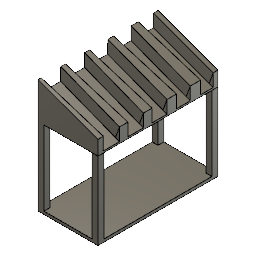
rail_interieur v3 (Autodesk Fusion 360 design; units mm, degrees)
Autodesk Fusion 360 part; units mm, degrees
note: some values were not read from the file. Chosen so that the rebuilt part matches the saved one: which pieces of a blend or face edit are solid.
sketch "Sketch1" plane through (0, 0, 0) normal (0, 0, 1) x (1, 0, 0)
  line L0 (0, 0) -> (100, 0)
  line L1 (100, 0) -> (100, 76)
  line L2 (100, 76) -> (0, 76)
  line L3 (0, 76) -> (0, 0)
  dimension "d17" = 76
  dimension "d18" = 100
  measures "d17" distance of L0.start
  measures "d18" distance of L0.start
extrude "Extrude1" add sketch "Sketch1" along normal blind 200
sketch "Sketch2" plane through (0, 0, 0) normal (0, 0, -1) x (-1, 0, 0)
  line L0 (0, 0) -> (0, 76)
  line L1 (0, 76) -> (-100, 76)
  line L2 (-100, 76) -> (-100, 0)
  line L3 (-100, 0) -> (0, 0)
  line L4 (0, 76) -> (0, 29.8312)
  line L5 (-100, 39.603) -> (0, 76)
  line L6 (-100, 39.603) -> (0, 29.8312)
  dimension "d21" = 70
  measures "d21" angle of L4 L5
extrude "Extrude2" cut sketch "Sketch2" against normal blind 200 contours L1 L2 L5
sketch "Sketch3" plane through (24.4259, 67.1097, 0) normal (0.34202, 0.939693, 0) x (0, 0, -1)
  line L0 (0, -80.4242) -> (0, 25.9935)
  line L1 (0, 25.9935) -> (-200, 25.9935)
  line L2 (-200, 25.9935) -> (-200, -80.4242)
  line L3 (-200, -80.4242) -> (0, -80.4242)
  line L4 (-194.57, 25.9935) -> (-162.27, 25.9935)
  line L5 (-164.07, -80.4242) -> (-162.27, 25.9935)
  line L6 (-194.57, 25.9935) -> (-191.07, -80.4242)
  line L7 (-164.07, -80.4242) -> (-191.07, -80.4242)
  line L8 (-154.33, 25.9935) -> (-122.33, 25.9935)
  line L9 (-124.2, -80.4242) -> (-122.33, 25.9935)
  line L10 (-154.33, 25.9935) -> (-150.2, -80.4242)
  line L11 (-113.93, 25.9935) -> (-83.93, 25.9935)
  line L12 (-84.95, -80.4242) -> (-109.95, -80.4242)
  line L13 (-113.93, 25.9935) -> (-109.95, -80.4242)
  line L14 (-83.93, 25.9935) -> (-84.95, -80.4242)
  line L15 (-69.2, -80.4242) -> (-73.98, 25.9935)
  line L16 (-73.98, 25.9935) -> (-44.98, 25.9935)
  line L17 (-44.98, 25.9935) -> (-46.2, -80.4242)
  line L18 (-69.2, -80.4242) -> (-46.2, -80.4242)
  line L19 (-29, -80.4242) -> (-32.78, 25.9935)
  line L20 (-7.78, 25.9935) -> (-32.78, 25.9935)
  line L21 (-7.78, 25.9935) -> (-8, -80.4242)
  line L22 (-29, -80.4242) -> (-8, -80.4242)
  dimension "d24" = 7.78
  dimension "d25" = 25
  dimension "d26" = 21
  dimension "d27" = 8
  dimension "d28" = 12.2
  dimension "d29" = 29
  dimension "d30" = 23
  dimension "d31" = 17.2
  dimension "d32" = 9.95
  dimension "d33" = 30
  dimension "d34" = 15.75
  dimension "d35" = 25
  dimension "d36" = 8.4
  dimension "d37" = 32
  dimension "d38" = 14.25
  dimension "d39" = 26
  dimension "d40" = 13.87
  dimension "d41" = 32.3
  dimension "d42" = 7.94
  dimension "d43" = 27
  measures "d24" distance of origin
  measures "d25" distance of origin
  measures "d26" distance of origin
  measures "d27" distance of origin
extrude "Extrude3" cut sketch "Sketch3" against normal blind 20 contours L1 L3 L19 L20 L21 L22 | L1 L3 L15 L16 L17 L18 | L1 L3 L11 L12 L13 L14 | L1 L3 L8 L9 L10 | L1 L3 L4 L5 L6 L7
extrude "Extrude4" cut 5 faces at (95.4397, 27.0737, 101.6167) (97.7199, 33.3384, 141.5333) (95.4397, 27.0737, 182.07) (97.7199, 33.3384, 53.8667) (97.7199, 33.3384, 22) along direction (0.939693, -0.34202, 0) blind 20
sketch "Sketch5" plane through (0, 0, 0) normal (0, 0, -1) x (-1, 0, 0)
  line L0 (0, 76) -> (-100, 39.603)
  line L1 (-100, 39.603) -> (-100, 0)
  line L2 (-100, 0) -> (0, 0)
  line L3 (0, 0) -> (0, 76)
  line L4 (-100, 0) -> (0, 0)
  line L5 (0, 0) -> (0, 15.3194)
  line L6 (0, 15.3194) -> (-100, 15.3194)
  line L7 (-100, 15.3194) -> (-100, 0)
  dimension "d48" = 3
extrude "Extrude5" cut sketch "Sketch5" against normal blind 200 contours L1 L2 L3 L4 L5 L6 L7
sketch "Sketch7" plane through (0, 0, 0) normal (0, 1, 0) x (1, 0, 0)
  line L0 (100, -8) -> (100, -29)
  line L1 (0, -7.78) -> (100, -8)
  circle A0 centre (110.5, -18.5231) radius 10.5
  line L2 (0, -44.98) -> (100, -46.2)
  line L3 (100, -46.2) -> (100, -69.2)
  circle A1 centre (111.5, -57.8412) radius 11.5
  line L4 (0, -83.93) -> (100, -84.95)
  line L5 (100, -84.95) -> (100, -109.95)
  circle A2 centre (112.5, -97.5782) radius 12.5
  line L6 (0, -122.33) -> (100, -124.2)
  line L7 (100, -124.2) -> (100, -150.2)
  circle A3 centre (113, -137.4454) radius 13
  line L8 (0, -162.27) -> (100, -164.07)
  line L9 (100, -164.07) -> (100, -191.07)
  circle A4 centre (113.5, -177.8152) radius 13.5
  circle A5 centre (113.5, -177.8152) radius 15.5
  circle A6 centre (113, -137.4454) radius 15
  circle A7 centre (112.5, -97.5782) radius 14.5
  circle A8 centre (111.5, -57.8412) radius 13.5
  circle A9 centre (110.5, -18.5231) radius 12.5
  dimension "d51" = 21
  dimension "d52" = 23
  dimension "d53" = 25
  dimension "d54" = 26
  dimension "d55" = 27
  dimension "d56" = 2
  dimension "d57" = 2
  dimension "d58" = 2
  dimension "d59" = 2
  dimension "d60" = 2
  measures "d51" diameter of A0
  measures "d52" diameter of A1
  measures "d53" diameter of A2
  measures "d54" diameter of A3
  measures "d55" diameter of A4
  measures "d56" distance of A4 A5
  measures "d57" distance of A3 A6
  measures "d58" distance of A2 A7
  measures "d59" distance of A1 A8
  measures "d60" distance of A0 A9
sketch "Sketch8" plane through (0, 0, 200) normal (0, 0, 1) x (1, 0, 0)
  line L0 (0, 15.3194) -> (100, 15.3194)
  line L1 (100, 15.3194) -> (100, 39.603)
  line L2 (100, 39.603) -> (0, 76)
  line L3 (0, 76) -> (0, 15.3194)
  line L4 (0, 95) -> (39.9891, 61.4452)
  line L5 (0, 76) -> (0, 95)
  line L6 (0, 76) -> (39.9891, 61.4452)
  dimension "d65" = 50
  measures "d65" angle of L4 L5
sketch "Sketch9" plane through (-2.5854, 0.941, 162.6631) normal (-0.015892, 0.005784, 0.999857) x (0.999874, 0, 0.015892)
  line L0 (2.5789, 75.0602) -> (2.5808, 53.7763)
  line L1 (2.5808, 53.7763) -> (95.7553, 19.8684)
  line L2 (95.7553, 19.8684) -> (102.5948, 38.6626)
  line L3 (102.5948, 38.6626) -> (2.5789, 75.0602)
  line L4 (3.1785, 93.8417) -> (43.1625, 60.2911)
  line L5 (3.1785, 74.842) -> (3.1785, 93.8417)
  line L6 (3.1785, 74.842) -> (43.1625, 60.2911)
sketch "Sketch17" plane through (100, 0, 0) normal (-1, 0, 0) x (0, 0, 1)
  line L0 (177.8152, -5) -> (177.8152, 15.319)
  line L1 (177.8152, 15.319) -> (170.1994, 15.319)
  line L2 (170.1994, 15.319) -> (170.1994, -5)
  line L3 (170.1994, -5) -> (177.8152, -5)
  line L4 (185.431, -5) -> (11.7408, -5)
  line L5 (11.7408, -5) -> (11.7408, 15.319)
  line L6 (11.7408, 15.319) -> (185.431, 15.319)
  line L7 (185.431, 15.319) -> (185.431, -5)
  line L8 (11.7408, -5) -> (11.7408, 15.319)
  line L9 (200, 15.3194) -> (0, 15.3194)
  line L10 (137.4454, -5) -> (137.4454, 15.319)
  line L11 (137.4454, 15.319) -> (129.9621, 15.319)
  line L12 (129.9621, 15.319) -> (129.9621, -5)
  line L13 (129.9621, -5) -> (137.4454, -5)
sketch "Sketch18" plane through (100, 0, 0) normal (1, 0, 0) x (0, 0, -1)
  line L0 (-185.431, -5) -> (-11.7408, -5)
  line L1 (-11.7408, 15.319) -> (-185.431, 15.319)
  line L2 (-129.9621, -5) -> (-129.9621, 15.319)
  line L3 (-122.4454, 15.319) -> (-152.4454, 15.319)
  line L4 (-144.9287, 15.319) -> (-144.9287, -5)
  line L5 (-152.4454, -5) -> (-122.4454, -5)
  line L6 (-170.1994, -5) -> (-170.1994, 15.319)
  line L7 (-162.3152, 15.319) -> (-193.3152, 15.319)
  line L8 (-185.431, 15.319) -> (-185.431, -5)
  line L9 (-193.3152, -5) -> (-162.3152, -5)
  line L10 (-90.2297, -5) -> (-90.2297, 15.319)
  line L11 (-83.0782, 15.319) -> (-112.0782, 15.319)
  line L12 (-104.9266, 15.319) -> (-104.9266, -5)
  line L13 (-112.0782, -5) -> (-83.0782, -5)
  line L14 (-50.7701, -5) -> (-50.7701, 15.319)
  line L15 (-44.3412, 15.319) -> (-71.3412, 15.319)
  line L16 (-64.9122, 15.319) -> (-64.9122, -5)
  line L17 (-71.3412, -5) -> (-44.3412, -5)
  line L18 (-11.7408, -5) -> (-11.7408, 15.319)
  line L19 (-6.0231, 15.319) -> (-31.0231, 15.319)
  line L20 (-25.3055, 15.319) -> (-25.3055, -5)
  line L21 (-31.0231, -5) -> (-6.0231, -5)
  line L22 (-162.3152, 15.319) -> (-152.4454, 15.319)
  line L23 (-152.4454, 15.319) -> (-152.4454, -5)
  line L24 (-152.4454, -5) -> (-162.3152, -5)
  line L25 (-162.3152, -5) -> (-162.3152, 15.319)
  line L26 (-122.4454, 15.319) -> (-112.0782, 15.319)
  line L27 (-112.0782, 15.319) -> (-112.0782, -5)
  line L28 (-112.0782, -5) -> (-122.4454, -5)
  line L29 (-122.4454, -5) -> (-122.4454, 15.319)
  line L30 (-83.0782, 15.319) -> (-71.3412, 15.319)
  line L31 (-71.3412, 15.319) -> (-71.3412, -5)
  line L32 (-71.3412, -5) -> (-83.0782, -5)
  line L33 (-83.0782, -5) -> (-83.0782, 15.319)
  line L34 (-44.3412, 15.319) -> (-31.0231, 15.319)
  line L35 (-31.0231, 15.319) -> (-31.0231, -5)
  line L36 (-31.0231, -5) -> (-44.3412, -5)
  line L37 (-44.3412, -5) -> (-44.3412, 15.319)
  line L38 (-11.7408, -5) -> (-11.7408, 15.319)
  line L39 (-185.431, 15.319) -> (-185.431, -5)
sketch "Sketch19" plane through (0, 0, 0) normal (0, 0, -1) x (-1, 0, 0)
  line L0 (-100, 15.3194) -> (0, 15.3194)
  line L1 (0, 15.3194) -> (0, 76)
  line L2 (0, 76) -> (-100, 39.603)
  line L3 (-100, 39.603) -> (-100, 15.3194)
  line L4 (-10, 72.3603) -> (0, 76)
  line L5 (0, -114) -> (-10, -114)
  line L6 (-10, -114) -> (-10, 72.3603)
  line L7 (0, 76) -> (0, -114)
  dimension "d83" = 190
  dimension "d85" = 10
extrude "Extrude15" add sketch "Sketch19" against normal blind 10 contours L0 L5 L6 L7
sketch "Sketch20" plane through (0, 0, 200) normal (0, 0, 1) x (1, 0, 0)
  line L0 (0, 15.3194) -> (100, 15.3194)
  line L1 (100, 15.3194) -> (100, 39.603)
  line L2 (100, 39.603) -> (0, 76)
  line L3 (0, 76) -> (0, 15.3194)
  line L4 (10, -114) -> (10, 15.3194)
  line L5 (10, 15.3194) -> (0, 15.3194)
  line L6 (0, 15.3194) -> (0, -114)
  line L7 (0, -114) -> (10, -114)
extrude "Extrude16" add sketch "Sketch20" against normal blind 10 contours L0 L4 L5 L6 L7
sketch "Sketch21" plane through (0, -114, 0) normal (0, -1, 0) x (1, 0, 0)
  line L0 (10, 200) -> (0, 200)
  line L1 (0, 200) -> (0, 190)
  line L2 (0, 190) -> (10, 190)
  line L3 (10, 190) -> (10, 200)
  line L4 (0, 200) -> (100, 200)
  line L5 (100, 200) -> (100, 0)
  line L6 (100, 0) -> (0, 0)
  line L7 (0, 0) -> (0, 200)
  line L8 (10, 0) -> (10, 10)
  line L9 (0, 10) -> (10, 10)
extrude "Extrude17" add sketch "Sketch21" against normal blind 5 contours L2 L3 L4 L5 L6 L7 L8 L9
sketch "Sketch22" plane through (0, -109, 0) normal (0, 1, 0) x (-1, 0, 0)
  line L0 (0, 10) -> (0, 190)
  line L1 (0, 190) -> (-10, 190)
  line L2 (-10, 190) -> (-10, 200)
  line L3 (-10, 200) -> (-100, 200)
  line L4 (-100, 200) -> (-100, 0)
  line L5 (-100, 0) -> (-10, 0)
  line L6 (-10, 0) -> (-10, 10)
  line L7 (-10, 10) -> (0, 10)
  line L8 (-100, 200) -> (-90, 200)
  line L9 (-90, 200) -> (-90, 190)
  line L10 (-90, 190) -> (-100, 190)
  line L11 (-100, 190) -> (-100, 200)
  line L12 (-100, 0) -> (-90, 0)
  line L13 (-90, 0) -> (-90, 10)
  line L14 (-90, 10) -> (-100, 10)
  line L15 (-100, 10) -> (-100, 0)
  dimension "d92" = 10
  dimension "d93" = 10
  dimension "d94" = 10
  dimension "d95" = 10
  measures "d94" distance of origin L14
extrude "Extrude18" add sketch "Sketch22" along normal blind 124.319 contours L4 L5 L12 L13 L14 L15 | L3 L4 L8 L9 L10 L11
sketch "Sketch23" plane through (0, 0, 0) normal (0, 0, -1) x (-1, 0, 0)
  line L0 (-100, 15.3194) -> (-10, 15.3194)
  line L1 (-10, 15.3194) -> (-10, -109)
  line L2 (-10, -109) -> (-90, -109)
  line L3 (-90, -109) -> (-90, 15.319)
  line L4 (-90, 15.319) -> (-100, 15.319)
  line L5 (-100, 15.319) -> (-100, -114)
  line L6 (-100, -114) -> (0, -114)
  line L7 (0, -114) -> (0, 76)
  line L8 (0, 76) -> (-100, 39.603)
  line L9 (-100, 39.603) -> (-100, 15.3194)
  line L10 (0, 54.7164) -> (-93.1596, 20.8091)
  line L11 (-82.5201, 15.319) -> (0, 50)
  line L12 (0, 15.3194) -> (-82.5201, 15.319)
  line L13 (0, 50) -> (0, 15.3194)
ref_plane "WorkPlane1" through (128.9986, 8.5909, 177.6099) normal (0.999912, 0, -0.013244) x (0.013244, 0, 0.999912)
sketch "Sketch28" plane through (128.9986, 8.5909, 177.6099) normal (0.999912, 0, -0.013244) x (0.013244, 0, 0.999912)
  line L0 (-169.3037, -6.7285) -> (-169.3037, 117.5909)
  line L1 (-169.1713, 117.5909) -> (-169.1713, -6.7285)
  line L2 (-169.3037, 23.5909) -> (-169.1713, 28.5909)
  line L3 (40.1619, 65.502) -> (40.0294, 60.502)
  line L4 (40.0294, 60.502) -> (-169.3037, 23.5909)
  line L5 (-169.1713, 28.5909) -> (40.1619, 65.502)
  line L6 (-146.8178, 13.5909) -> (-171.8178, 13.5909)
  dimension "d107" = 100
  dimension "d108" = 5
  dimension "d109" = 5
  dimension "d110" = 10
  measures "d107" angle of L1 L4
  measures "d110" distance of origin L6
extrude "Extrude23" add sketch "Sketch28" against normal blind 28.147 contours L1 L3 L4 L5
ref_plane "WorkPlane2" through (50, -64, 100) normal (0, -1, 0) x (1, 0, 0)
sketch "Sketch30" plane through (50, -64, 100) normal (0, -1, 0) x (1, 0, 0)
  line L0 (50, -90) -> (50, -91.1921)
  line L1 (50, -91.1921) -> (76.7581, -91.5465)
  line L2 (76.7581, -91.5465) -> (79.5306, 117.7683)
  line L3 (79.5306, 117.7683) -> (51.386, 118.1411)
  line L4 (51.386, 118.1411) -> (48.6291, -90)
  line L5 (48.6291, -90) -> (50, -90)
  line L6 (76.7581, -91.5465) -> (66.8905, -91.4158)
  line L7 (66.8905, -81.4158) -> (76.8905, -81.5465)
  line L8 (76.7581, -91.5465) -> (76.8905, -81.5465)
  line L9 (66.8905, -81.4158) -> (66.8905, -91.4158)
  line L10 (79.5306, 117.7683) -> (79.3999, 107.9007)
  line L11 (69.3999, 107.9007) -> (69.5323, 117.9007)
  line L12 (79.5306, 117.7683) -> (69.5323, 117.9007)
  line L13 (69.3999, 107.9007) -> (79.3999, 107.9007)
  line L14 (51.386, 118.1411) -> (51.2536, 108.1428)
  line L15 (51.2536, 108.1428) -> (61.2536, 108.0104)
  line L16 (61.2536, 118.0104) -> (51.386, 118.1411)
  line L17 (61.2536, 108.0104) -> (61.2536, 118.0104)
  dimension "d120" = 10
  dimension "d121" = 10
  dimension "d122" = 10
  dimension "d123" = 10
  dimension "d124" = 10
  dimension "d125" = 10
  dimension "d126" = 10
extrude "Extrude24" add sketch "Sketch30" along normal blind 50 and the other way up to surface contours L1 L2 L6 L7 L8 L9 | L3 L4 L14 L15 L16 L17 | L2 L3 L10 L11 L12 L13 second end surface through (126.7581, -20, 8.4535) normal (-0.0023, -0.984808, -0.173633) offset 0
sketch "Sketch32" plane through (126.6239, 0, -1.6772) normal (0.999912, 0, -0.013244) x (-0.013244, 0, -0.999912)
  line L0 (-10.1316, -114) -> (-10.1316, -15.0234)
  line L1 (-10.1316, -15.0234) -> (-219.3323, -51.9111)
  line L2 (-219.3323, -51.9111) -> (-219.4647, -56.9111)
  line L3 (-219.4647, -56.9111) -> (-219.4647, -114)
  line L4 (-219.4647, -114) -> (-209.5963, -114)
  line L5 (-209.5963, -114) -> (-209.5963, -55.171)
  line L6 (-209.5963, -55.171) -> (-20.1324, -21.7634)
  line L7 (-20.1324, -21.7634) -> (-20.1324, -114)
  line L8 (-20.1324, -114) -> (-10.1316, -114)
  line L9 (-219.3323, -51.9111) -> (-159.9903, -41.4475)
  line L10 (-191.3078, -109) -> (-191.3078, 15.319)
  line L11 (-11.3236, -15.2335) -> (-10.1316, -15.0234)
  line L12 (-10.1316, -15.0234) -> (-10.1316, -20)
  line L13 (-10.1316, -20) -> (-11.3236, -20.2102)
  line L14 (-11.3236, -20.2102) -> (-11.3236, -109)
  line L15 (-11.3236, -109) -> (-191.3078, -109)
  line L16 (-191.3078, -109) -> (-191.3078, 15.319)
  line L17 (-191.3078, 15.319) -> (-201.3069, 15.319)
  line L18 (-201.3069, 15.319) -> (-201.3069, -114)
  line L19 (-201.3069, -114) -> (-1.3244, -114)
  line L20 (-1.3244, -114) -> (-1.3244, 15.319)
  line L21 (-1.3244, 15.319) -> (-11.3236, 15.319)
  line L22 (-11.3236, 15.319) -> (-11.3236, -15.2335)
extrude "Extrude25" add sketch "Sketch32" along normal up to surface contours L1 L6 L9 L10 L16 L18 end surface through (100, -114, 200) normal (1, 0, 0) offset 0
delete_face "DeleteFace1" 1 faces at (119.1, -37.968, 138.692)
extrude "Extrude19" [suppressed]
extrude "Extrude20" [suppressed]
sketch "Sketch25" plane through (0, 0, 0) normal (0, 0, -1) x (-1, 0, 0)
  line L0 (-10.0002, 45.7972) -> (-10, 15.3194)
  line L1 (-10, 15.3194) -> (-10, -109)
  line L2 (-10, -109) -> (-90, -109)
  line L3 (-90, -109) -> (-90, 15.319)
  line L4 (-90, 15.319) -> (-100, 15.319)
  line L5 (-100, 15.319) -> (-100, -114)
  line L6 (-100, -114) -> (0, -114)
  line L7 (0, -114) -> (0, 15.3194)
  line L8 (0, 15.3194) -> (-0.0002, 47.5734)
  line L9 (-0.0002, 47.5734) -> (-5.7739, 47.5734)
  line L10 (-5.7739, 47.5734) -> (0, 50)
  line L11 (0, 50) -> (0, 76)
  line L12 (0, 76) -> (-100, 39.603)
  line L13 (-100, 39.603) -> (-100, 15.3194)
  line L14 (-100, 15.3194) -> (-82.5191, 15.3194)
  line L15 (-82.5191, 15.3194) -> (-10.0002, 45.7972)
  line L16 (-5.7739, 47.5734) -> (0, 50)
  line L17 (0, 50) -> (-0.0002, 47.5734)
  line L18 (-0.0002, 47.5734) -> (-5.7739, 47.5734)
sketch "Sketch26" plane through (0, 0, 190) normal (0, 0, -1) x (-1, 0, 0)
  line L0 (-10, 15.3194) -> (-10, -109)
  line L1 (-10, -109) -> (0, -109)
  line L2 (0, -109) -> (0, 15.3194)
  line L3 (0, 15.3194) -> (-0.0002, 47.5734)
  line L4 (-0.0002, 47.5734) -> (-5.7739, 47.5734)
  line L5 (-5.7739, 47.5734) -> (-10.0002, 45.7972)
  line L6 (-10.0002, 45.7972) -> (-10, 15.3194)
  line L7 (-0.0002, 47.5734) -> (-5.7739, 47.5734)
  line L8 (-5.7739, 47.5734) -> (0, 50)
  line L9 (0, 50) -> (-0.0002, 47.5734)
extrude "Extrude21" [suppressed]
extrude "Extrude22" [suppressed]
sketch "Sketch27" plane through (100, 0, 0) normal (1, 0, 0) x (0, 0, -1)
  line L0 (-200, -114) -> (0, -114)
  line L1 (0, -114) -> (0, 15.319)
  line L2 (0, 15.319) -> (-10, 15.319)
  line L3 (-10, 15.319) -> (-10, -109)
  line L4 (-10, -109) -> (-190, -109)
  line L5 (-190, -109) -> (-190, 15.319)
  line L6 (-190, 15.319) -> (-200, 15.319)
  line L7 (-200, 15.319) -> (-200, -114)
sketch "Sketch11" plane through (-2.0269, 0.7377, 122.7489) normal (-0.01651, 0.006009, 0.999846) x (0.999864, 0, 0.01651)
  line L0 (2.0197, 75.2636) -> (2.0218, 53.9797)
  line L1 (2.0218, 53.9797) -> (95.1975, 20.0718)
  line L2 (95.1975, 20.0718) -> (102.0369, 38.8659)
  line L3 (102.0369, 38.8659) -> (2.0197, 75.2636)
  line L4 (3.3021, 93.7966) -> (43.2857, 60.2464)
  line L5 (3.3021, 74.797) -> (3.3021, 93.7966)
  line L6 (3.3021, 74.797) -> (43.2857, 60.2464)
sketch "Sketch12" plane through (-0.7581, 0.2759, 84.1714) normal (-0.009006, 0.003278, 0.999954) x (0.999959, 0, 0.009006)
  line L0 (0.7559, 75.7245) -> (0.7565, 54.4408)
  line L1 (0.7565, 54.4408) -> (93.9209, 20.5333)
  line L2 (93.9209, 20.5333) -> (100.761, 39.3273)
  line L3 (100.761, 39.3273) -> (0.7559, 75.7245)
  line L4 (1.8013, 94.3439) -> (41.7888, 60.7904)
  line L5 (1.8013, 75.344) -> (41.7888, 60.7904)
  line L6 (1.8013, 75.344) -> (1.8013, 94.3439)
sketch "Sketch13" plane through (-0.4877, 0.1775, 45.272) normal (-0.010772, 0.003921, 0.999934) x (0.999942, 0, 0.010772)
  line L0 (0.4845, 75.8231) -> (0.4854, 54.5394)
  line L1 (0.4854, 54.5394) -> (93.6519, 20.6318)
  line L2 (93.6519, 20.6318) -> (100.4919, 39.4258)
  line L3 (100.4919, 39.4258) -> (0.4845, 75.8231)
  line L4 (2.1544, 94.2152) -> (42.1412, 60.6623)
  line L5 (2.1544, 75.2153) -> (2.1544, 94.2152)
  line L6 (2.1544, 75.2153) -> (42.1412, 60.6623)
sketch "Sketch14" plane through (-0.0152, 0.0055, 7.8337) normal (-0.001943, 0.000707, 0.999998) x (0.999998, 0, 0.001943)
  line L0 (0.0151, 75.9945) -> (0.0151, 54.7109)
  line L1 (0.0151, 54.7109) -> (93.175, 20.8036)
  line L2 (93.175, 20.8036) -> (100.0154, 39.5974)
  line L3 (100.0154, 39.5974) -> (0.0151, 75.9945)
  line L4 (0.3885, 94.8586) -> (40.3776, 61.3038)
  line L5 (0.3885, 75.8586) -> (0.3885, 94.8586)
  line L6 (0.3885, 75.8586) -> (40.3776, 61.3038)
extrude "Extrude7" [suppressed]
extrude "Extrude8" [suppressed]
extrude "Extrude9" [suppressed]
extrude "Extrude10" [suppressed]
extrude "Extrude11" [suppressed]
extrude "Extrude12" [suppressed]
